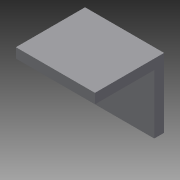
# Autodesk Inventor part: BumperStop
Saved by Autodesk Inventor 2013 (Build 170138000, 138)
## iProperties
Created: 2014-01-29
Part Number: BumperStop
Material: Generic
Document SubType Name: Modeling
Designer: 215152
Density: 1 g/cm^3
Author: 215152
Autodesk Inventor part; units mm, degrees
ref_plane "YZ Plane" through (0, 0, 0) normal (1, 0, 0) x (0, 1, 0)
ref_plane "XZ Plane" through (0, 0, 0) normal (0, 1, 0) x (-1, 0, 0)
ref_plane "XY Plane" through (0, 0, 0) normal (0, 0, 1) x (1, 0, 0)
sketch "Sketch1" plane through (0, 0, 0) normal (1, 0, 0) x (0, 1, 0)
  line L0 (0, 0) -> (19.05, 0)
  line L1 (19.05, 0) -> (19.05, 19.05)
  line L2 (19.05, 19.05) -> (0, 19.05)
  line L3 (0, 19.05) -> (0, 0)
  line L4 (19.05, 19.05) -> (22.225, 19.05)
  line L5 (22.225, 19.05) -> (22.225, -3.175)
  line L6 (22.225, -3.175) -> (19.05, -3.175)
  line L7 (19.05, -3.175) -> (19.05, 19.05)
  line L8 (19.05, -3.175) -> (0, -3.175)
  line L9 (0, -3.175) -> (0, 0)
  line L10 (0, 0) -> (19.05, 0)
  line L11 (19.05, 0) -> (19.05, -3.175)
  dimension "d0" = 19.05
  dimension "d1" = 19.05
  dimension "d2" = 3.175
  dimension "d3" = 22.225
  constraints: 24 end point, 6 parallel, 3 horizontal, 3 perpendicular
  measures "d0" distance of L2.end L1.end
  measures "d1" distance of L1.end L0.end
  measures "d2" distance of L5.end L6.end
  measures "d3" distance of L4.end L5.end
extrude "Extrusion1" add sketch "Sketch1" along normal blind 25.4 contours L0 L7 L8 L9 | L1 L4 L5 L6 L7
body "Solid1"
